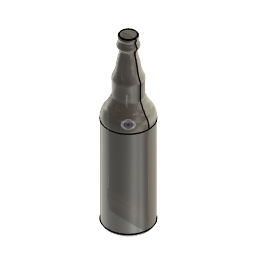
Glass Bottle (Autodesk Fusion 360 design; units mm, degrees)
part number: 2026-02-08-22-51-25-885
part number: 2026-02-10-11-10-00-833
Autodesk Fusion 360 part; units mm, degrees
sketch "Sketch1" plane through (0, 0, 0) normal (0, 1, 0) x (1, 0, 0) in component "beer bottle "
  line L0 (0, -116.343203) -> (0, 125)
  line L1 (0, 125) -> (30, 125)
  line L2 (30, 125) -> (30, -9)
  spline S0 degree 5 poles (30, -9) (30.070745, -9.109035) (30.197857, -9.35577) (30.34539, -9.811867) (30.455817, -10.592027) (30.450604, -11.844583) (30.304039, -13.34617) (30.019968, -15.039682) (29.605082, -16.830028) (29.069181, -18.573743) (28.428433, -20.127679) (27.704944, -21.38004) (26.934813, -22.319227) (26.156502, -23.016012) (25.445736, -23.81023) (24.823722, -24.940922) (24.223605, -26.298947) (23.571737, -27.690619) (22.830456, -28.918716) (22.046623, -29.920606) (21.431511, -30.942228) (20.990185, -32.051949) (20.640741, -33.241277) (20.261577, -34.446175) (19.758721, -35.594034) (19.141346, -36.647747) (18.524367, -37.619738) (18.037939, -38.552435) (17.785796, -39.504182) (17.733043, -40.542053) (17.756554, -41.707757) (17.804471, -43.000459) (17.835803, -44.399031) (17.837786, -45.870799) (17.810585, -47.384805) (17.765846, -48.926057) (17.720279, -50.494437) (17.692372, -52.094421) (17.697873, -53.728026) (17.7457, -55.385745) (17.833888, -57.039893) (17.944961, -58.633238) (18.043224, -60.079547) (18.084904, -61.299681) (18.026118, -62.275048) (17.833047, -63.050513) (17.487961, -63.861926) (17.006932, -64.896211) (16.432455, -66.178396) (15.82023, -67.66713) (15.227845, -69.268957) (14.703682, -70.884372) (14.273147, -72.447224) (13.936896, -73.937324) (13.679206, -75.362698) (13.473355, -76.751108) (13.288408, -78.13736) (13.094942, -79.553345) (12.872345, -81.014652) (12.611255, -82.517133) (12.310271, -84.045061) (11.974171, -85.576237) (11.611449, -87.088518) (11.232319, -88.565286) (10.846097, -90.002465) (10.460346, -91.411416) (10.088788, -92.807112) (9.75502, -94.200112) (9.503576, -95.58423) (9.394753, -96.932512) (9.540183, -98.173114) (9.949408, -99.252726) (10.559108, -100.146618) (11.264109, -100.864319) (11.945625, -101.456119) (12.502118, -102.023219) (12.856676, -102.677116) (12.961679, -103.499911) (12.805826, -104.492045) (12.414631, -105.576359) (11.846737, -106.648525) (11.19059, -107.612055) (10.562915, -108.424174) (10.100399, -109.123273) (9.913517, -109.783216) (10.051404, -110.481113) (10.449596, -111.252349) (10.955778, -112.092704) (11.386971, -112.978521) (11.576862, -113.881208) (11.426501, -114.783869) (10.994422, -115.499152) (10.487669, -116.030502) (10.068647, -116.382461) (9.838841, -116.557873) knots 0 0 0 0 0 0 0.01111111 0.02222222 0.03333333 0.04444444 0.05555556 0.06666667 0.07777778 0.08888889 0.1 0.11111111 0.12222222 0.13333333 0.14444444 0.15555556 0.16666667 0.17777778 0.18888889 0.2 0.21111111 0.22222222 0.23333333 0.24444444 0.25555556 0.26666667 0.27777778 0.28888889 0.3 0.31111111 0.32222222 0.33333333 0.34444444 0.35555556 0.36666667 0.37777778 0.38888889 0.4 0.41111111 0.42222222 0.43333333 0.44444444 0.45555556 0.46666667 0.47777778 0.48888889 0.5 0.51111111 0.52222222 0.53333333 0.54444444 0.55555556 0.56666667 0.57777778 0.58888889 0.6 0.61111111 0.62222222 0.63333333 0.64444444 0.65555556 0.66666667 0.67777778 0.68888889 0.7 0.71111111 0.72222222 0.73333333 0.74444444 0.75555556 0.76666667 0.77777778 0.78888889 0.8 0.81111111 0.82222222 0.83333333 0.84444444 0.85555556 0.86666667 0.87777778 0.88888889 0.9 0.91111111 0.92222222 0.93333333 0.94444444 0.95555556 0.96666667 0.97777778 0.98888889 1 1 1 1 1 1
  line L3 (28.965671, -20.144958) -> (15.972211, -38.604635)
  line L4 (32, -17) -> (20.368573, -29.055494)
  line L5 (20, -56.000001) -> (15.649516, -69.935434)
  line L6 (19.184571, -30.293442) -> (16.464945, -48.890554)
  line L7 (10, -85.000001) -> (8.930459, -107.811664)
  line L8 (0, -116.343203) -> (10.107515, -116.343203)
  point P0 (30, -15)
  point P1 (26.184287, -23.027747)
  point P2 (22.468941, -29.374797)
  point P3 (20, -35)
  point P4 (17.824758, -39.591998)
  point P5 (17.824758, -46.403466)
  point P6 (17.824758, -56.775474)
  point P7 (17.824758, -62.967718)
  point P8 (15, -70)
  point P9 (13.180576, -78.912745)
  point P10 (11.322903, -88.20111)
  point P11 (9.46523, -96.405832)
  point P12 (11.322903, -100.895209)
  point P13 (12.870963, -103.062494)
  point P14 (11.322903, -107.397065)
  point P15 (10, -110)
  point P16 (11.322903, -112.970084)
  point P17 (9.838841, -116.557873)
  point P18 (30, -15)
  point P19 (26.184287, -23.027747)
  point P20 (22.468941, -29.374797)
  point P21 (20, -35)
  point P22 (17.824758, -39.591998)
  point P23 (17.824758, -46.403466)
  point P24 (17.824758, -56.775474)
  point P25 (17.824758, -62.967718)
  point P26 (15, -70)
  point P27 (13.180576, -78.912745)
  point P28 (11.322903, -88.20111)
  point P29 (9.46523, -96.405832)
  point P30 (11.322903, -100.895209)
  point P31 (12.870963, -103.062494)
  point P32 (11.322903, -107.397065)
  point P33 (10, -110)
  point P34 (11.322903, -112.970084)
  dimension "d3" = 30
  dimension "d4" = 134
  constraint vertical L0
  constraint perpendicular L0 L1
  constraint perpendicular L1 L2
  constraint coincident P18 P0
  constraint coincident P21 P3
  constraint coincident P26 P8
  constraint coincident P33 P15
  constraint perpendicular L0 L8
  measures "d3" distance of L0.end L1.end
  measures "d4" distance of L1.end L2.end
revolve "Revolve1" add sketch "Sketch1" angle 360 about axis through (0, 0, 116.343203) along (0, 0, -1) in component "beer bottle "
fillet "Fillet1" radius 5 1 edges at (-27.96982, -10.848463, -125) in component "beer bottle "
fillet "Fillet2" radius 1 1 edges at (-9.423512, -3.655033, 116.343203) in component "beer bottle "
sketch "Sketch2" plane through (0, 0, 0) normal (0, 0, 1) x (1, 0, 0) in component "beer bottle "
  circle A0 centre (0, 0) radius 7
  dimension "d10" = 14
  constraint coincident A0.centre origin
  measures "d10" diameter of A0
component "beer bottle " placed x (1, 0, 0) y (0, 1, 0) z (0, 0, 1) at (0, 0, 0)
